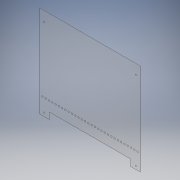
# Autodesk Inventor part: Lateral Acrilico
Saved by Autodesk Inventor 2018 (Build 220112000, 112)
## iProperties
Created: 2018-07-06
Part Number: Lateral Acrilico
Material: PMMA plástico
Document SubType Name: Chapa de metal
Designer: Regner
Density: 1.188 g/cm^3
Sheet Metal Rule: Padrão_mm
Appearance: Policarbonato - Transparente
Author: Regner
Autodesk Inventor part; units mm, degrees
ref_plane "YZ Plane" through (0, 0, 0) normal (1, 0, 0) x (0, 1, 0)
ref_plane "XZ Plane" through (0, 0, 0) normal (0, 1, 0) x (-1, 0, 0)
ref_plane "XY Plane" through (0, 0, 0) normal (0, 0, 1) x (1, 0, 0)
sketch "Esboço2" plane through (0, 0, 0) normal (0, 1, 0) x (-1, 0, 0)
  line L0 (-153.4, 150) -> (153.4, 150)
  line L1 (153.4, 150) -> (153.4, -150)
  line L2 (153.4, -150) -> (-153.4, -150)
  line L3 (-153.4, -150) -> (-153.4, 150)
  line L4 (-153.4, 150) -> (153.4, -150) construction
  line L5 (153.4, 150) -> (-153.4, -150) construction
  point P0 (0, 0)
  dimension "d2" = 306.8
  dimension "d3" = 300
  measures "d2" distance of L1.end L2.end
  measures "d3" distance of L0.end L1.end
extrude "Placa1" add sketch "Esboço2" along normal blind 0.5
sketch "Esboço3" plane through (0, 0.5, 0) normal (0, 1, 0) x (1, 0, 0)
  line L0 (153.4, -150) -> (-153.4, -150) projected
  line L1 (-153.4, -150) -> (-153.4, 150) projected
  point P0 (0, 0)
  point P1 (-140, -120)
  point P2 (140, -120)
  point P3 (-140, 120)
  point P4 (140, 120)
  dimension "d5" = 120
  dimension "d6" = 140
  dimension "d9" = 280
  dimension "d12" = 240
  constraints: 1 horizontal, 1 vertical, 3 other
  measures "d5" vertical distance of point (0, 0) point (-140, -120)
  measures "d6" horizontal distance of point (0, 0) point (-140, -120)
  measures "d9" distance of point (-140, -120) point (140, -120)
  measures "d12" distance of point (-140, -120) point (-140, 120)
hole "Furo1" at (-140, 0.5, 120) at (140, 0.5, 120) at (-140, 0.5, -120) at (140, 0.5, -120) direction (0, -1, 0) diameter 4 end through all
sketch "Esboço4" plane through (0, 0, 0) normal (0, -1, 0) x (1, 0, 0)
  circle A0 centre (-140, -120) radius 2 projected
  circle A1 centre (-140, 120) radius 2 projected
  circle A2 centre (140, 120) radius 2 projected
  circle A3 centre (140, -120) radius 2 projected
  line L0 (153.4, 150) -> (-153.4, 150) projected
  line L1 (-153.4, 150) -> (-153.4, -150) projected
  line L2 (-153.4, -150) -> (153.4, -150) projected
  line L3 (153.4, -150) -> (153.4, 150) projected
  line L4 (-153.4, -150) -> (153.4, -150) projected
  line L5 (-123.4, -150) -> (123.4, -150)
  line L6 (123.4, -130) -> (123.4, -110)
  line L7 (123.4, -110) -> (-123.4, -110)
  line L8 (-123.4, -110) -> (-123.4, -130)
  line L9 (-153.4, 150) -> (-153.4, -150) projected
  line L10 (-153.4, -150) -> (-123.4, -150)
  line L11 (-123.4, -130) -> (-153.4, -130)
  line L12 (-153.4, -130) -> (-153.4, -150)
  line L13 (153.4, -150) -> (153.4, 150) projected
  line L14 (123.4, -150) -> (153.4, -150)
  line L15 (153.4, -150) -> (153.4, -130)
  line L16 (153.4, -130) -> (123.4, -130)
  point P0 (0, 0)
  dimension "d22" = 30
  dimension "d23" = 30
  dimension "d24" = 40
  dimension "d27" = 20
  dimension "d30" = 246.8
  constraints: 20 end point, 4 parallel, 3 horizontal, 3 point on line, 2 perpendicular, 1 collinear
  measures "d22" distance between parallel lines of L3 L6
  measures "d23" distance between parallel lines of L1 L8
  measures "d24" distance between parallel lines of L2 L7
  measures "d27" distance between parallel lines of L2 L11
  measures "d30" distance of L6.end L7.end
extrude "Extrusão2" cut sketch "Esboço4" against normal through all contours L3 L2 L1 L11 L8 L7 L6 L16
sketch "Esboço5" plane through (0, 0, 0) normal (0, -1, 0) x (1, 0, 0)
  line L0 (153.4, -130) -> (153.4, 150) projected
  line L1 (-153.4, 150) -> (-153.4, -130) projected
  circle A0 centre (-145, -80) radius 2.5
  line L2 (-153.4, -130) -> (-123.4, -130) projected
  point P0 (0, 0)
  dimension "d31" = 306.8
  dimension "d32" = 5
  dimension "d33" = 8.4
  dimension "d34" = 50
  constraints: 1 centre point
  measures "d31" distance between parallel lines of L0 L1
  measures "d32" diameter of A0
  measures "d33" distance from line of L1 A0.centre
  measures "d34" distance from line of L2 A0.centre
extrude "Extrusão3" cut sketch "Esboço5" against normal up to surface (0.5 mm away)
pattern_linear "Padrão retangular1" count 30 spacing 10 along (1, 0, 0) of "Extrusão3"
equation "\"d9\" = 2 * d6"
equation "\"d12\" = 2 * d5"
equation "\"d20\" = Espessura"
equation "\"d4\" = Espessura"
equation "\"Raio_vergadura\" = Espessura"
equation "\"Largura_alívio_de_vergadura\" = Espessura"
equation "\"Profundidade_alívio_de_vergadura\" = 0.5 * Espessura"
equation "\"Tamanho_alívio_de_dobra\" = 4 * Espessura"
equation "\"Remanescente_mínimo\" = 2 * Espessura"
equation "\"Raiodetransição\" = Raio_vergadura"
equation "\"Tamanho_de_raio_de_Jacobi\" = Raio_vergadura"
equation "\"TamanhoFolga\" = Espessura"
equation "\"Espessura\" = 0.5"
